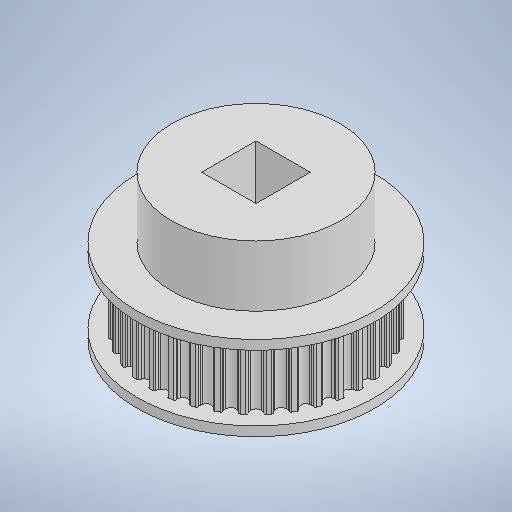
# Autodesk Inventor part: Driven pulley 36
Saved by Autodesk Inventor 2025.2 (Build 292293000, 293)
## iProperties
Created: 2025-02-03
Part Number: Driven pulley 36
Material: Generic
Document SubType Name: Modeling
Designer: caomi
Density: 1 g/cm^3
Appearance: Default
Author: caomi
Autodesk Inventor part; units mm, degrees
ref_plane "YZ Plane" through (0, 0, 0) normal (1, 0, 0) x (0, 1, 0)
ref_plane "XZ Plane" through (0, 0, 0) normal (0, 1, 0) x (-1, 0, 0)
ref_plane "XY Plane" through (0, 0, 0) normal (0, 0, 1) x (1, 0, 0)
sketch "Sketch1" plane through (0, 0, 0) normal (0, 1, 0) x (-1, 0, 0)
  circle A0 centre (0, 0) radius 11.4592 construction
  circle A1 centre (0, 0) radius 10.4552 construction
  line L0 (0, 0) -> (11.4592, 0) construction
  line L1 (0, 0) -> (11.4156, -0.9987) construction
  line L2 (0, 0) -> (11.3737, -1.3965) construction
  circle A2 centre (0, 0) radius 11.2052 construction
  line L3 (0, 0) -> (10.4552, 0) construction
  arc A3 (10.6691, -0.4922) -> (10.4154, -0.9112) centre (10.9683, -0.9596) ccw
  arc A4 (11.062, -0.3673) -> (10.861, -0.4001) centre (11.1216, -1.3656) ccw
  circle A5 centre (0, 0) radius 11.0552 construction
  arc A6 (11.203, -0.2206) -> (11.2052, 0) centre (0, 0) ccw
  line L4 (0, 0) -> (11.203, -0.2206) construction
  line L5 (0, 0) -> (11.2052, 0) construction
  arc A7 (11.062, -0.3673) -> (11.203, -0.2206) centre (11.053, -0.2176) ccw
  arc A8 (10.861, -0.4001) -> (10.6691, -0.4922) centre (11.0131, -0.9635) ccw
  arc A9 (10.4154, 0.9112) -> (10.6691, 0.4922) centre (10.9683, 0.9596) ccw
  arc A10 (10.861, 0.4001) -> (11.062, 0.3673) centre (11.1216, 1.3656) ccw
  arc A11 (11.2052, 0) -> (11.203, 0.2206) centre (0, 0) ccw
  arc A12 (11.203, 0.2206) -> (11.062, 0.3673) centre (11.053, 0.2176) ccw
  arc A13 (10.6691, 0.4922) -> (10.861, 0.4001) centre (11.0131, 0.9635) ccw
  arc A14 (10.4154, -0.9112) -> (10.4154, 0.9112) centre (0, 0) ccw
  circle A15 centre (0, 0) radius 10.4552
  circle A16 centre (0, 0) radius 11.4592
  circle A17 centre (0, 0) radius 12.7
  point P0 (10.4154, -0.9112)
  dimension "d0" = 22.9183
  dimension "d1" = 5
  dimension "d2" = 2
  dimension "d4" = 1.004
  dimension "d13" = 0.75
  dimension "d14" = 0.555
  dimension "d15" = 1
  dimension "d16" = 0.15
  dimension "d35" = 25.4
  constraints: 33 point on circle, 17 centre point, 12 end point, 10 coincident, 9 symmetric about line, 6 point on line, 3 tangent, 1 concentric, 1 horizontal, 8 other
  measures "d0" diameter of A0
  measures "d1" angle of L0 L1
  measures "d2" angle of L2 L1
  measures "d4" radial gap between concentric circles of A0 A1
  measures "d13" radial gap between concentric circles of A1 A2
  measures "d14" radius of A3
  measures "d15" radius of A4
  measures "d16" radial gap between concentric circles of A5 A2
  measures "d35" diameter of A17
extrude "Extrusion1" add sketch "Sketch1" along normal blind 4.5 contours A3 A14 A9 A13 A10 A12 A11 A6 A7 A4 A8 | A15 A14 | A16 | A17
extrude "Extrusion2" cut sketch "Sketch1" along normal blind 3.5 contours A3 A14 A9 A13 A10 A12 A11 A6 A7 A4 A8 | A16 | A17
extrude "Extrusion3" add sketch "Sketch1" along normal blind 3.5 contours A3 A14 A9 A13 A10 A12 A11 A6 A7 A4 A8
pattern_circular "Circular Pattern1" count 36 over 360 about axis through (0, 0, 0) along (0, 1, 0) of "Extrusion3"
mirror "Mirror3" about plane through (0, 0, 0) normal (0, -1, 0)
sketch "Sketch2" plane through (0, 4.5, 0) normal (0, 1, 0) x (1, 0, 0)
  line L0 (2.9, 2.9) -> (-2.9, 2.9)
  line L1 (-2.9, 2.9) -> (-2.9, -2.9)
  line L2 (-2.9, -2.9) -> (2.9, -2.9)
  line L3 (2.9, -2.9) -> (2.9, 2.9)
  line L4 (2.9, 2.9) -> (-2.9, -2.9) construction
  line L5 (-2.9, 2.9) -> (2.9, -2.9) construction
  circle A0 centre (0, 0) radius 12.7 projected
  dimension "d37" = 5.8
  dimension "d38" = 5.8
  constraints: 12 end point, 2 coincident, 2 midpoint, 2 parallel, 1 horizontal, 1 perpendicular
  measures "d37" distance of L2.end L0.start
  measures "d38" distance of L0.start L0.end
extrude "Extrusion4" cut sketch "Sketch2" against normal through all contours L3 L2 L1 L0
sketch "Sketch3" plane through (0, 3.5, 0) normal (0, -1, 0) x (1, 0, 0)
  circle A0 centre (0, 0) radius 9
  circle A1 centre (0, 0) radius 11.4592 projected
  line L0 (2.9, 2.9) -> (2.9, -2.9) projected
  line L1 (2.9, -2.9) -> (-2.9, -2.9) projected
  line L2 (-2.9, 2.9) -> (2.9, 2.9) projected
  line L3 (-2.9, -2.9) -> (-2.9, 2.9) projected
  dimension "d36" = 18
  constraints: 1 centre point, 1 coincident
  measures "d36" diameter of A0
extrude "Extrusion5" add sketch "Sketch3" against normal blind 7.5 contours A0
equation "\"d0\" = PulleyDia"
equation "\"d1\" = 0.5 * ToothAng"
equation "\"d2\" = TransOffsetAngle"
equation "\"d4\" = PLD + ToothHeight"
equation "\"d13\" = ToothHeight"
equation "\"d14\" = Root_Radius"
equation "\"d15\" = TransRadius"
equation "\"d16\" = Shoulder_Radius"
equation "\"d38\" = d37"
equation "\"ToothPitch\" = 2"
equation "\"TransOffsetAngle\" = 0.2 * ToothAng"
equation "\"Shoulder_Radius\" = 0.15"
equation "\"Root_Radius\" = 0.555"
equation "\"TransRadius\" = 1"
equation "\"ToothHeight\" = 0.75"
equation "\"PLD\" = 0.254"
equation "\"PulleyDia\" = 22.918312"
equation "\"ToothAng\" = 10deg"
body "Solid1"
